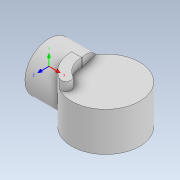
# Autodesk Inventor part: hip_inventor
Saved by Autodesk Inventor 2020 (Build 240168000, 168)
## iProperties
Created: 2021-01-07
Part Number: hip_inventor
Material: Generic
Document SubType Name: Modeling
Designer: DELL
Density: 1 g/cm^3
Appearance: Default
Author: DELL
Autodesk Inventor part; units mm, degrees
ref_plane "YZ Plane" through (0, 0, 0) normal (1, 0, 0) x (0, 1, 0)
ref_plane "XZ Plane" through (0, 0, 0) normal (0, 1, 0) x (-1, 0, 0)
ref_plane "XY Plane" through (0, 0, 0) normal (0, 0, 1) x (1, 0, 0)
sketch "Sketch1" plane through (0, 0, 0) normal (1, 0, 0) x (0, 1, 0)
  circle A0 centre (0, 0) radius 28
  line L0 (-14.5, -23.953079) -> (-14.5, 23.953079)
  line L1 (14.5, -23.953079) -> (14.5, 23.953079)
  line L2 (0, -28) -> (0, 28) construction
  dimension "d0" = 56
  dimension "d19" = 29
  constraints: 6 end point, 6 point on circle, 3 vertical, 1 centre point, 1 coincident, 1 midpoint, 1 other
  measures "d0" diameter of A0
  measures "d19" distance between parallel lines of L1 L0
extrude "Extrusion1" add sketch "Sketch1" along normal blind 66 contours A0 L1 | L0 A0
sketch "Sketch2" plane through (0, 0, 0) normal (0, 1, 0) x (-1, 0, 0)
  line L0 (-66, 23.953079) -> (-66, -23.953079)
  circle A0 centre (-66, 0) radius 39.5
  point P0 (0, 0)
  dimension "d3" = 79
  constraints: 1 centre point, 1 midpoint
  measures "d3" diameter of A0
extrude "Extrusion2" add sketch "Sketch2" along normal mid plane 56
sketch "Sketch3" plane through (0, 0, 0) normal (0, 1, 0) x (-1, 0, 0)
  circle A0 centre (-66, 0) radius 39.5 projected
  circle A1 centre (-66, 0) radius 31.5
  circle A2 centre (-66, 0) radius 39.5
  point P0 (0, 0)
  point P1 (-26.5, 0)
  dimension "d12" = 79
  dimension "d13" = 63
  constraints: 2 centre point, 2 coincident, 1 horizontal alignment
  measures "d12" diameter of A2
  measures "d13" diameter of A1
sketch "Sketch4" plane through (66, 28, 0) normal (0, 1, 0) x (1, 0, 0)
  circle A0 centre (0, 0) radius 39.5
  circle A1 centre (0, 0) radius 28
  circle A2 centre (-33.75, 0) radius 5.75
  circle A3 centre (-16.875, -29.228357) radius 5.75
  line L0 (0, 0) -> (-16.875, -29.228357) construction
  line L1 (0, 0) -> (-33.75, 0) construction
  line L2 (-34.371506, 23.953079) -> (-39.5, 23.953079)
  line L3 (-66, 23.953079) -> (-31.408598, 23.953079)
  line L4 (-66, 23.953079) -> (-31.408598, 23.953079)
  line L5 (-31.408598, 23.953079) -> (-34.371506, 23.953079)
  point P0 (-66, 0)
  point P1 (-39.5, 0)
  point P2 (-66, 0)
  point P3 (-66, 0)
  point P4 (-28, 0)
  point P5 (-14, -24.248711)
  point P6 (-19.75, -34.208003)
  point P7 (-28.059354, 0.824045)
  point P8 (-39.5, 0)
  dimension "d20" = 56
  dimension "d21" = 60
  constraints: 8 end point, 2 centre point, 2 coincident, 2 collinear, 2 horizontal, 2 tangent, 1 horizontal alignment, 1 point on line, 5 other
  measures "d20" diameter of A1
  measures "d21" angle of L1 L0
extrude "Extrusion5" add sketch "Sketch1" along normal up to surface contours L1 A0 L0 round surface about axis through (66, 0, 0) along (0, 1, 0) radius 39.5 far side no
extrude "Extrusion3" cut sketch "Sketch4" against normal blind 10.5 contours A0 A3 A1 A2 | A1 picked at (-31.227253, 11.780989)
sketch "Sketch6" plane through (0, 28, 0) normal (0, 1, 0) x (1, 0, 0)
  arc A0 (38, 0) -> (26.5, 0) centre (32.25, 0) ccw
  circle A1 centre (32.25, 0) radius 5.75
  line L0 (33.098632, 21.857493) -> (26.5, 21.857493)
  line L1 (26.5, 21.857493) -> (26.5, 0)
  circle A2 centre (66, 0) radius 39.5
  line L2 (33.098632, 21.857493) -> (37.852244, 1.295128)
  arc A3 (38, 0) -> (26.5, 0) centre (32.25, 0) ccw
  arc A4 (38, 0) -> (52, -24.248711) centre (66, 0) ccw
  circle A5 centre (32.25, 0) radius 5.75
  point P0 (0, 0)
  point P1 (37.852244, 1.295128)
  constraints: 6 end point, 2 coincident, 2 tangent, 1 horizontal, 1 horizontal alignment, 1 perpendicular, 6 other
extrude "Extrusion7" add sketch "Sketch6" against normal up to surface (10.5 mm away) contours A0 A2 L2 | L1 L0 A2
sketch "Sketch5" plane through (0, 0, 0) normal (-1, 0, 0) x (0, 0, 1)
  circle A0 centre (0, 0) radius 28
  line L0 (-21.857493, 17.5) -> (-21.857493, 28)
  line L1 (0, 28) -> (-1.295128, 28)
  line L2 (-21.857493, 28) -> (0, 28)
  point P0 (34.208003, 17.5)
  constraints: 4 end point, 1 horizontal, 1 point on circle, 1 vertical
extrude "Extrusion6" cut sketch "Sketch5" against normal through all contours A0 L0 L2 L1
body "Solid1"
